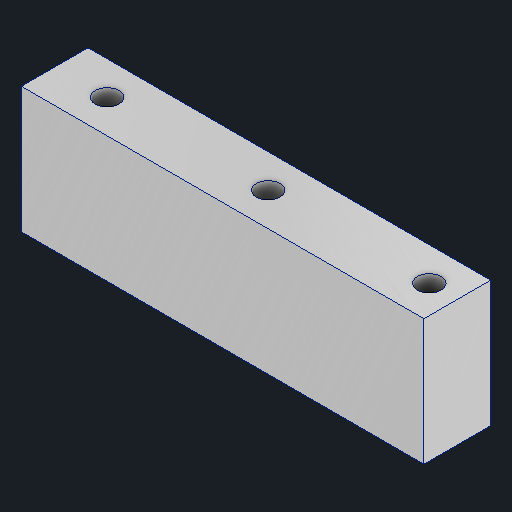
# Autodesk Inventor part: Drive Frame Spacing Block
Saved by Autodesk Inventor 2025.1 (Build 291241020, 241B)
## iProperties
Created: 2025-05-06
Part Number: Drive Frame Spacing Block
Material: Aluminum 6061
Document SubType Name: Modeling
Designer: Joshua Eah
Density: 2.7 g/cm^3
Appearance: Aluminum - Flat
Mass: 34.1639 g
Surface Area: 45.1055 cm^2
Volume: 12.6533 cm^3
Author: Joshua Eah
Autodesk Inventor part; units mm, degrees
ref_plane "YZ Plane" through (0, 0, 0) normal (1, 0, 0) x (0, 1, 0)
ref_plane "XZ Plane" through (0, 0, 0) normal (0, 1, 0) x (-1, 0, 0)
ref_plane "XY Plane" through (0, 0, 0) normal (0, 0, 1) x (1, 0, 0)
sketch "Sketch1" plane through (0, 0, 0) normal (0, 1, 0) x (-1, 0, 0)
  line L0 (0, 0) -> (-57.5, 0)
  line L1 (-57.5, 0) -> (-57.5, -9.525)
  line L2 (-57.5, -9.525) -> (0, -9.525)
  line L3 (0, -9.525) -> (0, 0)
  line L4 (0, -4.7625) -> (-57.5, -4.7625) construction
  circle A0 centre (-7.493, -4.7625) radius 1.5
  circle A1 centre (-53.5, -4.7625) radius 1.5
  circle A2 centre (-30.4927, -4.7625) radius 1.5
  dimension "d0" = 9.525
  dimension "d1" = 57.5
  dimension "d2" = 3
  dimension "d3" = 7.493
  dimension "d4" = 4
  dimension "d14" = 22.9997
  dimension "d15" = 23.0073
  constraints: 10 end point, 3 centre point, 3 point on line, 2 equal radius, 2 midpoint, 2 parallel, 1 horizontal, 1 perpendicular
  measures "d0" distance of L1.end L0.end
  measures "d1" distance of L1.end L2.end
  measures "d2" diameter of A0
  measures "d3" distance from line of A0.centre L3
  measures "d4" distance from line of L1 A1.centre
  measures "d14" distance of A2.centre A0.centre
  measures "d15" distance of A1.centre A2.centre
extrude "Extrusion1" add sketch "Sketch1" along normal blind 18 contours L3 L2 L1 L0 | A0 | A1 | A2
hole "Hole1" at (53.5, 0, -4.7625) at (7.493, 0, -4.7625) at (30.4927, 0, -4.7625) direction (0, 1, 0) diameter 3.4036 end through all clearance for "Flat Head Machine Screw" size "M3" standard "Ansi Metric M Profile"
body "Solid1"
